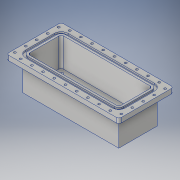
# Autodesk Inventor part: Electronics Box
Saved by Autodesk Inventor 2017 (Build 210142000, 142)
## iProperties
Created: 2017-02-16
Part Number: Electronics Box
Material: Aluminum 6061
Document SubType Name: Modeling
Designer: qupec
Density: 2.7 g/cm^3
Appearance: Aluminum - Flat
Mass: 270.39 g
Surface Area: 483.635 cm^2
Volume: 100.145 cm^3
Author: qupec
Autodesk Inventor part; units mm, degrees
ref_plane "YZ Plane" through (0, 0, 0) normal (1, 0, 0) x (0, 1, 0)
ref_plane "XZ Plane" through (0, 0, 0) normal (0, 1, 0) x (-1, 0, 0)
ref_plane "XY Plane" through (0, 0, 0) normal (0, 0, 1) x (1, 0, 0)
sketch "Sketch1" plane through (0, 0, 0) normal (0, 1, 0) x (-1, 0, 0)
  line L0 (63.5, 25.4) -> (-63.5, 25.4)
  line L1 (-63.5, 25.4) -> (-63.5, -25.4)
  line L2 (-63.5, -25.4) -> (63.5, -25.4)
  line L3 (63.5, -25.4) -> (63.5, 25.4)
  point P0 (0, 0)
  dimension "d0" = 50.8
  dimension "d1" = 25.4
  dimension "d2" = 63.5
  dimension "d3" = 127
  constraints: 8 end point, 2 parallel, 1 horizontal, 1 perpendicular
  measures "d0" distance between parallel lines of L2 L0
  measures "d1" distance from line of point (0, 0) L0
  measures "d2" distance from line of point (0, 0) L1
  measures "d3" distance of L0.start L0.end
extrude "Extrusion1" add sketch "Sketch1" along normal blind 6.35
sketch "Sketch2" plane through (0, 6.35, 0) normal (0, 1, 0) x (1, 0, 0)
  line L0 (-60.325, -22.225) -> (60.325, -22.225)
  line L1 (60.325, -22.225) -> (60.325, 22.225)
  line L2 (60.325, 22.225) -> (-60.325, 22.225)
  line L3 (-60.325, 22.225) -> (-60.325, -22.225)
  line L4 (-63.5, -25.4) -> (63.5, -25.4) projected
  line L5 (63.5, -25.4) -> (63.5, 25.4) projected
  line L6 (63.5, 25.4) -> (-63.5, 25.4) projected
  line L7 (-63.5, 25.4) -> (-63.5, -25.4) projected
  point P0 (0, 0)
  dimension "d6" = 3.175
  dimension "d7" = 3.175
  dimension "d8" = 3.175
  dimension "d9" = 3.175
  constraints: 8 end point, 2 parallel, 1 horizontal, 1 perpendicular
  measures "d6" distance between parallel lines of L7 L3
  measures "d7" distance between parallel lines of L4 L0
  measures "d8" distance between parallel lines of L5 L1
  measures "d9" distance between parallel lines of L6 L2
extrude "Extrusion2" add sketch "Sketch2" along normal blind 38.1
fillet "Fillet1" radius 3.175 4 edges at (-60.325, 25.4, -22.225) (60.325, 25.4, -22.225) (60.325, 25.4, 22.225) (-60.325, 25.4, 22.225)
sketch "Sketch4" plane through (63.5, 0, -25.4) normal (0, 0, -1) x (-1, 0, 0)
  line L0 (127, 0) -> (127, 44.45) projected
  line L1 (127, 44.45) -> (104.775, 44.45)
  line L2 (104.775, 44.45) -> (104.775, 38.1)
  line L3 (104.775, 38.1) -> (127, 38.1)
  line L4 (127, 38.1) -> (127, 44.45)
  line L5 (74.6125, 44.45) -> (52.3875, 44.45)
  line L6 (52.3875, 44.45) -> (52.3875, 38.1)
  line L7 (52.3875, 38.1) -> (74.6125, 38.1)
  line L8 (74.6125, 38.1) -> (74.6125, 44.45)
  line L9 (22.225, 44.45) -> (0, 44.45)
  line L10 (0, 44.45) -> (0, 38.1)
  line L11 (0, 38.1) -> (22.225, 38.1)
  line L12 (22.225, 38.1) -> (22.225, 44.45)
  point P0 (63.5, 0)
  dimension "d28" = 22.225
  dimension "d29" = 6.35
  dimension "d32" = 52.3875
  constraints: 24 end point, 2 horizontal, 2 parallel, 1 collinear, 1 perpendicular, 15 other
  measures "d28" distance of L3.end L2.end
  measures "d29" distance between parallel lines of L1 L3
  measures "d32" distance of L2.end L6.end
extrude "Extrusion4" [suppressed]
sketch "Sketch5" plane through (-63.5, 0, -25.4) normal (-1, 0, 0) x (0, 0, 1)
  line L0 (-15.24, 38.1) -> (0, 22.86)
  line L1 (0, 0) -> (0, 44.45) projected
  line L2 (0, 44.45) -> (0, 38.1) projected
  line L3 (0, 22.86) -> (0, 38.1)
  line L4 (0, 38.1) -> (-15.24, 38.1)
  point P0 (25.4, 0)
  dimension "d39" = 15.24
  constraints: 6 end point, 1 perpendicular, 1 point on line, 1 vertical
  measures "d39" distance of L2.end L0.end
extrude "Extrusion5" [suppressed]
pattern_linear "Rectangular Pattern1" [suppressed]
pattern_linear "Rectangular Pattern2" [suppressed]
sketch "Sketch6" plane through (-60.325, 38.1, -40.64) normal (0, -1, 0) x (1, 0, 0)
  line L0 (123.825, 15.24) -> (-3.175, 15.24) projected
  line L1 (15.875, 0) -> (0, 0) projected
  line L2 (15.875, 0) -> (15.875, 15.24) projected
  line L3 (0, 15.24) -> (0, 0) projected
  point P0 (60.325, 40.64)
  point P1 (7.9375, 7.62)
  point P2 (60.3377, 7.62)
  point P3 (112.7379, 7.62)
  dimension "d48" = 7.62
  dimension "d49" = 15.24
  dimension "d50" = 15.875
  dimension "d51" = 7.9375
  dimension "d54" = 52.4002
  constraints: 1 horizontal, 2 other
  measures "d48" distance from line of L0 point (7.938, 7.62)
  measures "d49" distance between parallel lines of L0 L1
  measures "d50" distance between parallel lines of L2 L3
  measures "d51" distance from line of point (7.938, 7.62) L3
  measures "d54" distance of point (7.938, 7.62) point (60.338, 7.62)
hole "Hole1" [suppressed]
fillet "Fillet2" [suppressed]
fillet "Fillet3" [suppressed]
mirror "Mirror1" [suppressed]
fillet "Fillet4" [suppressed]
sketch "Sketch13" plane through (0, 44.45, 0) normal (0, 1, 0) x (1, 0, 0)
  line L0 (-74.295, 36.195) -> (74.295, 36.195)
  line L1 (74.295, 36.195) -> (74.295, -36.195)
  line L2 (74.295, -36.195) -> (-74.295, -36.195)
  line L3 (-74.295, -36.195) -> (-74.295, 36.195)
  line L4 (63.5, 25.4) -> (-63.5, 25.4) projected
  line L5 (-63.5, 25.4) -> (-63.5, -25.4) projected
  line L6 (-63.5, -25.4) -> (63.5, -25.4) projected
  line L7 (63.5, -25.4) -> (63.5, 25.4) projected
  point P0 (0, 0)
  dimension "d81" = 10.795
  dimension "d82" = 10.795
  dimension "d83" = 10.795
  dimension "d84" = 10.795
  constraints: 8 end point, 2 parallel, 1 horizontal, 1 perpendicular
  measures "d81" distance between parallel lines of L4 L0
  measures "d82" distance between parallel lines of L5 L3
  measures "d83" distance between parallel lines of L6 L2
  measures "d84" distance between parallel lines of L1 L7
extrude "Extrusion12" add sketch "Sketch13" against normal blind 6.35
fillet "Fillet5" radius 3.175 8 edges at (63.5, 38.1, 0) (0, 38.1, -25.4) (-63.5, 38.1, 0) (0, 38.1, 25.4) (-74.295, 41.275, 36.195) (-74.295, 41.275, -36.195) (74.295, 41.275, 36.195) (74.295, 41.275, -36.195)
sketch "Sketch14" plane through (0, 38.1, 0) normal (0, -1, 0) x (1, 0, 0)
  line L0 (71.12, 36.195) -> (-71.12, 36.195) projected
  line L1 (66.675, 28.575) -> (-66.675, 28.575) projected
  line L2 (74.295, -33.02) -> (74.295, 33.02) projected
  line L3 (74.295, -33.02) -> (74.295, 33.02) projected
  line L4 (74.295, 0) -> (-74.2494, 0) construction
  line L5 (71.12, -36.195) -> (-71.12, -36.195)
  line L6 (66.675, -28.575) -> (66.675, 28.575) projected
  line L7 (-71.12, -36.195) -> (71.12, -36.195) projected
  line L8 (0, -36.195) -> (0, 36.195) construction
  point P0 (0, 0)
  point P1 (59.2667, 32.385)
  point P2 (44.45, 32.385)
  point P3 (29.6333, 32.385)
  point P4 (14.8167, 32.385)
  point P5 (0, 32.385)
  point P6 (-14.8167, 32.385)
  point P7 (-29.6333, 32.385)
  point P8 (-44.45, 32.385)
  point P9 (-59.2667, 32.385)
  point P10 (59.2667, -32.385)
  point P11 (44.45, -32.385)
  point P12 (29.6333, -32.385)
  point P13 (14.8167, -32.385)
  point P14 (0, -32.385)
  point P15 (-14.8167, -32.385)
  point P16 (-29.6333, -32.385)
  point P17 (-44.45, -32.385)
  point P18 (-59.2667, -32.385)
  point P19 (70.485, -28.956)
  point P20 (70.485, -14.478)
  point P21 (70.485, 0)
  point P22 (70.485, 14.478)
  point P23 (70.485, 28.956)
  point P24 (-70.485, -28.956)
  point P25 (-70.485, -14.478)
  point P26 (-70.485, 0)
  point P27 (-70.485, 14.478)
  point P28 (-70.485, 28.956)
  dimension "d88" = 3.81
  dimension "d89" = 7.62
  dimension "d94" = 14.8167
  dimension "d99" = 118.5333
  dimension "d100" = 59.2667
  dimension "d101" = 7.62
  dimension "d102" = 3.81
  dimension "d103" = 7.239
  dimension "d106" = 14.478
  dimension "d128" = 57.912
  dimension "d129" = 28.956
  constraints: 16 symmetric about line, 6 end point, 3 midpoint, 2 horizontal, 1 vertical, 12 other
  measures "d88" distance from line of L0 point (59.267, 32.385)
  measures "d89" distance between parallel lines of L0 L1
  measures "d94" distance of point (59.267, 32.385) point (44.45, 32.385)
  measures "d99" distance of point (-59.267, 32.385) point (59.267, 32.385)
  measures "d100" horizontal distance of point (0, 0) point (59.267, 32.385)
  measures "d101" distance between parallel lines of L2 L6
  measures "d102" distance from line of L2 point (70.485, -28.956)
  measures "d103" distance from line of point (70.485, -28.956) L5
  measures "d106" distance of point (70.485, -28.956) point (70.485, -14.478)
  measures "d128" distance of point (70.485, -28.956) point (70.485, 28.956)
  measures "d129" distance from line of L4 point (70.485, -28.956)
hole "Hole2" at (59.2667, 38.1, 32.385) at (44.45, 38.1, 32.385) at (29.6333, 38.1, 32.385) at (14.8167, 38.1, 32.385) at (0, 38.1, 32.385) at (-14.8167, 38.1, 32.385) at (-29.6333, 38.1, 32.385) at (-44.45, 38.1, 32.385) at (-59.2667, 38.1, 32.385) at (-59.2667, 38.1, -32.385) at (-44.45, 38.1, -32.385) at (-29.6333, 38.1, -32.385) at (-14.8167, 38.1, -32.385) at (0, 38.1, -32.385) at (14.8167, 38.1, -32.385) at (29.6333, 38.1, -32.385) at (44.45, 38.1, -32.385) at (59.2667, 38.1, -32.385) at (70.485, 38.1, -28.956) at (70.485, 38.1, -14.478) at (70.485, 38.1, 0) at (70.485, 38.1, 14.478) at (70.485, 38.1, 28.956) at (-70.485, 38.1, 28.956) at (-70.485, 38.1, 14.478) at (-70.485, 38.1, 0) at (-70.485, 38.1, -14.478) at (-70.485, 38.1, -28.956) direction (0, 1, 0) diameter 2.9464 depth 25.4 tip angle 118
sketch "Sketch17" plane through (0, 0, 0) normal (0, -1, 0) x (1, 0, 0)
  line L0 (50.4, -14.25) -> (43.6, -14.25) projected
  line L1 (43.6, -14.25) -> (43.6, 9.75) projected
  line L2 (43.6, 9.75) -> (50.4, 9.75) projected
  line L3 (50.4, 9.75) -> (50.4, -14.25) projected
  point P0 (0, 0)
extrude "Extrusion14" cut sketch "Sketch17" against normal blind 6.35
sketch "Sketch18" plane through (0, 0, 0) normal (0, -1, 0) x (1, 0, 0)
  line L0 (59.29, -7.85) -> (52.49, -7.85) projected
  line L1 (52.49, -7.85) -> (52.49, 5.95) projected
  line L2 (52.49, 5.95) -> (59.29, 5.95) projected
  line L3 (59.29, 5.95) -> (59.29, -7.85) projected
  line L4 (-56.75, -4.3) -> (-49.95, -4.3) projected
  line L5 (-49.95, -4.3) -> (-49.95, -14.2) projected
  line L6 (-49.95, -14.2) -> (-56.75, -14.2) projected
  line L7 (-56.75, -14.2) -> (-56.75, -4.3) projected
  point P0 (0, 0)
extrude "Extrusion15" cut sketch "Sketch18" against normal through all
sketch "Sketch19" plane through (0, 0, 0) normal (0, -1, 0) x (1, 0, 0)
  circle A0 centre (55.89, 8.15) radius 1.6 projected
  circle A1 centre (55.89, -10.05) radius 1.6 projected
  circle A2 centre (-53.35, -2.1) radius 1.6 projected
  circle A3 centre (-53.35, -16.4) radius 1.6 projected
  circle A4 centre (47, -16.4) radius 1.6 projected
  circle A5 centre (47, 11.9) radius 1.6 projected
  point P0 (0, 0)
extrude "Extrusion16" cut sketch "Sketch19" against normal through all
sketch "Sketch20" plane through (0, 44.45, 0) normal (0, 1, 0) x (1, 0, 0)
  circle A0 centre (47, 16.4) radius 1.6 projected
  circle A1 centre (-53.35, 2.1) radius 1.6 projected
  circle A2 centre (55.89, -8.15) radius 1.6 projected
  circle A3 centre (55.89, 10.05) radius 1.6 projected
  circle A4 centre (-53.35, 16.4) radius 1.6 projected
  circle A5 centre (47, -11.9) radius 1.6 projected
  line L0 (-56.75, 4.3) -> (-56.75, 14.2) projected
  line L1 (-56.75, 14.2) -> (-49.95, 14.2) projected
  line L2 (-49.95, 14.2) -> (-49.95, 4.3) projected
  line L3 (-49.95, 4.3) -> (-56.75, 4.3) projected
  line L4 (59.29, 7.85) -> (59.29, -5.95) projected
  line L5 (59.29, -5.95) -> (52.49, -5.95) projected
  line L6 (52.49, -5.95) -> (52.49, 7.85) projected
  line L7 (52.49, 7.85) -> (59.29, 7.85) projected
  line L8 (50.4, 14.25) -> (50.4, -9.75) projected
  line L9 (50.4, -9.75) -> (43.6, -9.75) projected
  line L10 (43.6, -9.75) -> (43.6, 14.25) projected
  line L11 (43.6, 14.25) -> (50.4, 14.25) projected
  arc A6 (-60.325, -19.05) -> (-57.15, -22.225) centre (-57.15, -19.05) ccw projected
  line L12 (-57.15, -22.225) -> (57.15, -22.225) projected
  arc A7 (57.15, -22.225) -> (60.325, -19.05) centre (57.15, -19.05) ccw projected
  line L13 (60.325, -19.05) -> (60.325, 19.05) projected
  arc A8 (60.325, 19.05) -> (57.15, 22.225) centre (57.15, 19.05) ccw projected
  line L14 (57.15, 22.225) -> (-57.15, 22.225) projected
  arc A9 (-57.15, 22.225) -> (-60.325, 19.05) centre (-57.15, 19.05) ccw projected
  line L15 (-60.325, 19.05) -> (-60.325, -19.05) projected
  line L16 (-57.15, 24.9809) -> (57.15, 24.9809)
  arc A10 (63.0809, 19.05) -> (57.15, 24.9809) centre (57.15, 19.05) ccw
  line L17 (63.0809, 19.05) -> (63.0809, -19.05)
  arc A11 (57.15, -24.9809) -> (63.0809, -19.05) centre (57.15, -19.05) ccw
  line L18 (57.15, -24.9809) -> (-57.15, -24.9809)
  arc A12 (-63.0809, -19.05) -> (-57.15, -24.9809) centre (-57.15, -19.05) ccw
  line L19 (-63.0809, -19.05) -> (-63.0809, 19.05)
  arc A13 (-57.15, 24.9809) -> (-63.0809, 19.05) centre (-57.15, 19.05) ccw
  line L20 (57.15, 28.1559) -> (-57.15, 28.1559)
  arc A14 (-57.15, 28.1559) -> (-66.2559, 19.05) centre (-57.15, 19.05) ccw
  line L21 (-66.2559, 19.05) -> (-66.2559, -19.05)
  arc A15 (-66.2559, -19.05) -> (-57.15, -28.1559) centre (-57.15, -19.05) ccw
  line L22 (-57.15, -28.1559) -> (57.15, -28.1559)
  arc A16 (57.15, -28.1559) -> (66.2559, -19.05) centre (57.15, -19.05) ccw
  line L23 (66.2559, -19.05) -> (66.2559, 19.05)
  arc A17 (66.2559, 19.05) -> (57.15, 28.1559) centre (57.15, 19.05) ccw
  point P0 (0, 0)
  dimension "d130" = 2.7559
  dimension "d131" = 3.175
  constraints: 16 end point, 16 point on circle, 8 centre point, 14 other
  measures "d130" distance between parallel lines of L14 L16
  measures "d131" distance between parallel lines of L16 L20
extrude "Extrusion18" cut sketch "Sketch20" against normal blind 2.032 contours A17 L23 A16 L22 A15 L21 A14 L20
equation "\"d1\" = 0.5 * d0"
equation "\"d2\" = 0.5 * d3"
equation "\"d7\" = d6"
equation "\"d8\" = d6"
equation "\"d9\" = d6"
equation "\"d48\" = 0.5 * d49"
equation "\"d51\" = 0.5 * d50"
equation "\"d81\" = d83"
equation "\"d82\" = d83"
equation "\"d84\" = d83"
equation "\"d88\" = 0.5 * d89"
equation "\"d100\" = 0.5 * d99"
equation "\"d102\" = 0.5 * d101"
equation "\"d129\" = 0.5 * d128"
body "Solid1"
